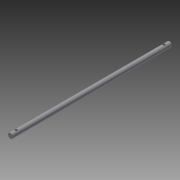
# Autodesk Inventor part: metal_shaft
Saved by Autodesk Inventor 2015 (Build 190159000, 159)
## iProperties
Created: 2017-09-26
Part Number: metal_shaft
Material: Generic
Document SubType Name: Modeling
Designer: Anshul
Density: 1 g/cm^3
Appearance: Default
Author: Anshul
Autodesk Inventor part; units mm, degrees
ref_plane "YZ Plane" through (0, 0, 0) normal (1, 0, 0) x (0, 1, 0)
ref_plane "XZ Plane" through (0, 0, 0) normal (0, 1, 0) x (-1, 0, 0)
ref_plane "XY Plane" through (0, 0, 0) normal (0, 0, 1) x (1, 0, 0)
sketch "Sketch1" plane through (0, 0, 0) normal (0, 1, 0) x (-1, 0, 0)
  line L0 (0, 0) -> (0, -200)
  line L1 (0, 0) -> (6.3, 0)
  line L2 (6.3, 0) -> (6.3, -200)
  line L3 (6.3, -200) -> (0, -200)
  line L4 (3.15, 0) -> (3.15, -200)
  line L5 (3.15, 0) -> (3.15, -7)
  line L6 (3.15, -200) -> (3.15, -193)
  circle A0 centre (3.15, -193) radius 1.5
  circle A1 centre (3.15, -7) radius 1.5
  dimension "d0" = 200
  dimension "d1" = 6.3
  dimension "d2" = 7
  dimension "d3" = 7
  dimension "d4" = 3
  dimension "d5" = 3
  constraints: 14 end point, 2 centre point, 2 coincident, 2 midpoint, 2 perpendicular, 2 point on line, 1 horizontal, 1 vertical
  measures "d0" distance of L0.start L0.end
  measures "d1" distance of L0.start L1.end
  measures "d2" distance of L4.start L5.end
  measures "d3" distance of L4.end L6.end
  measures "d4" diameter of A0
  measures "d5" diameter of A1
revolve "Revolution1" add sketch "Sketch1" angle 360 about axis through (-3.15, 0, 0) along (0, 0, -1)
extrude "Extrusion1" cut sketch "Sketch1" along normal mid plane 10 contours A1 L4 | L4 A1 | A0 L4 | L4 A0
body "Solid1"
